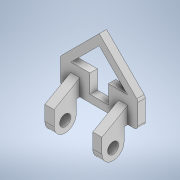
# Autodesk Inventor part: 01-1
Saved by Autodesk Inventor 2022 (Build 260153000, 153)
## iProperties
Created: 2021-09-12
Part Number: 01-1
Material: 일반
Document SubType Name: Modeling
Designer: 서울공업고등학교
Density: 1 g/cm^3
Appearance: 기본값
Author: 서울공업고등학교
Autodesk Inventor part; units mm, degrees
ref_plane "XZ Plane" through (0, 0, 0) normal (0, 1, 0) x (-1, 0, 0)
ref_plane "XY Plane" through (0, 0, 0) normal (0, 0, 1) x (1, 0, 0)
sketch "스케치1" plane through (0, 0, 0) normal (0, 0, 1) x (1, 0, 0)
  line L0 (0, 0) -> (0, 40)
  line L1 (0, 0) -> (40, 0) construction
  line L2 (0, 0) -> (-21, 0)
  line L3 (-15.3431, 14) -> (-5, 14)
  line L4 (-5, 14) -> (-5, 4)
  line L5 (-5, 4) -> (0, 4)
  line L6 (-21, 0) -> (-21, 14)
  line L7 (-21, 14) -> (0, 35)
  line L8 (-15.3431, 14) -> (0, 29.3431)
  line L9 (0, 0) -> (21, 0)
  line L10 (15.3431, 14) -> (5, 14)
  line L11 (5, 14) -> (5, 4)
  line L12 (5, 4) -> (0, 4)
  line L13 (21, 0) -> (21, 14)
  line L14 (21, 14) -> (0, 35)
  line L15 (15.3431, 14) -> (0, 29.3431)
  dimension "d0" = 40
  dimension "d2" = 35
  dimension "d3" = 4
  dimension "d4" = 10
  dimension "d6" = 42
  dimension "d8" = 4
  dimension "d9" = 10
  dimension "d10" = 45
  constraints: 32 end point, 5 symmetric about line, 4 point on line, 3 perpendicular, 2 vertical, 1 horizontal, 1 parallel
  measures "d0" distance of L0.start L0.end
  measures "d2" distance of L0.start L7.end
  measures "d3" distance between parallel lines of L2 L5
  measures "d4" diameter of L4 L0
  measures "d6" diameter of L6 L0
  measures "d8" distance between parallel lines of L8 L7
  measures "d9" distance between parallel lines of L5 L3
  measures "d10" angle of L0 L7
extrude "돌출1" add sketch "스케치1" against normal blind 4 contours L2 L6 L7 L0 L8 L3 L4 L5 | L0 L12 L11 L10 L15 L14 L13 L9
ref_plane "작업 평면1" through (10.5, 0, 0) normal (1, 0, 0) x (0, 1, 0)
sketch "스케치3" plane through (10.5, 0, 0) normal (1, 0, 0) x (0, 1, 0)
  circle A0 centre (-7, 8) radius 3
  arc A1 (-7, 14) -> (-7, 2) centre (-7, 8) ccw
  line L0 (14, 0) -> (0, 0) projected
  line L1 (9, 0) -> (1, 14)
  line L2 (1, 14) -> (-7, 14)
  line L3 (0, 0) -> (0, -4) projected
  line L4 (0, 0) -> (0, 2)
  line L5 (0, 2) -> (-7, 2)
  dimension "d14" = 6
  dimension "d15" = 12
  dimension "d16" = 8
  dimension "d17" = 8
  dimension "d18" = 6
  dimension "d19" = 12
  dimension "d20" = 14
  dimension "d21" = 7
  constraints: 8 end point, 2 centre point, 2 perpendicular, 2 point on circle, 1 coincident, 1 point on line, 1 tangent, 1 vertical
  measures "d14" diameter of A0
  measures "d15" diameter of A1
  measures "d16" horizontal distance of L1.end L1.start
  measures "d17" horizontal distance of A0.centre L1.end
  measures "d18" distance of L3.end L4.end
  measures "d19" vertical distance of L3.end A0.centre
  measures "d20" vertical distance of L1.start L1.end
  measures "d21" distance from line of L3 A0.centre
extrude "돌출2" add sketch "스케치3" along normal blind 5
mirror "미러1" about plane through (0, 0, 0) normal (1, 0, 0) of "돌출2"
fillet "모깎기1" radius 2 4 edges at (-21, 14, -2) (-21, 0, -2) (21, 14, -2) (21, 0, -2)
